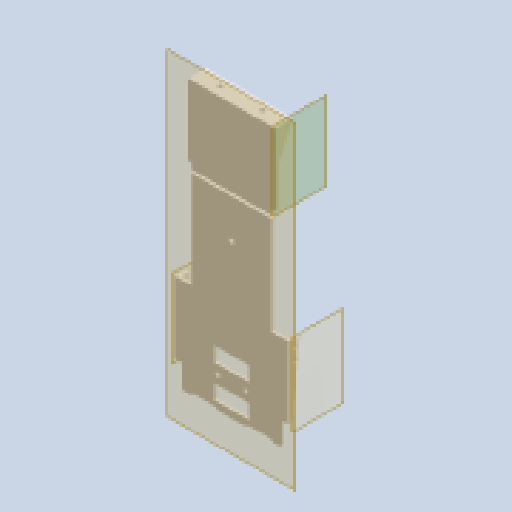
# Autodesk Inventor part: Деталь1
Saved by Autodesk Inventor 2024.2 (Build 282272000, 272)
## iProperties
Created: 2025-10-10
Part Number: Деталь1
Material: Типовые
Document SubType Name: Modeling
Designer: katya_notebook
Density: 1 g/cm^3
Appearance: По умолчанию
Author: katya_notebook
Autodesk Inventor part; units mm, degrees
ref_plane "YZ Plane" through (0, 0, 0) normal (1, 0, 0) x (0, 1, 0)
ref_plane "XZ Plane" through (0, 0, 0) normal (0, 1, 0) x (-1, 0, 0)
ref_plane "XY Plane" through (0, 0, 0) normal (0, 0, 1) x (1, 0, 0)
ref_plane "РабПлоскость1" through (46.6, -88.9135, 41) normal (0, 0, 1) x (1, 0, 0)
sketch "Эскиз1" plane through (46.6, -88.9135, 41) normal (0, 0, 1) x (1, 0, 0)
  line L0 (-9.7, 217.1229) -> (-9.7, 156.7629) projected
  line L1 (-83.5, 217.1229) -> (-9.7, 217.1229) projected
  line L2 (-83.5, 156.7629) -> (-83.5, 217.1229) projected
  line L3 (-80.1, 156.7629) -> (-83.5, 156.7629) projected
  line L4 (-80.1, 152.0768) -> (-80.1, 156.7629) projected
  line L5 (-9.7, 156.7629) -> (-13.1, 156.7629) projected
  line L6 (-13.1, 156.7629) -> (-13.1, 152.0768) projected
  line L7 (-13.1, 152.0768) -> (-80.1, 152.0768) projected
  line L8 (-13.1, 149.4521) -> (-13.1, 152.6229) projected
  line L9 (-13.1, 149.4521) -> (-13.1, 67.1229) projected
  line L10 (-80.1, 152.6229) -> (-80.1, 149.4521) projected
  line L11 (-80.1, 67.1229) -> (-80.1, 149.4521) projected
  line L12 (-13.1, 58.2834) -> (-13.1, 67.1229) projected
  line L13 (-13.1, 67.1229) -> (1.3, 67.1229) projected
  line L14 (1.3, 67.1229) -> (1.3, 6.7629) projected
  line L15 (1.3, 6.7629) -> (-4.4, 6.7629) projected
  line L16 (-4.4, 6.7629) -> (-4.4, -10.0571) projected
  arc A0 (-7.4, -13.0571) -> (-4.4, -10.0571) centre (-7.4, -10.0571) ccw projected
  line L17 (-7.4, -13.0571) -> (-10.4431, -13.0571) projected
  arc A1 (-11.7002, -12.6127) -> (-10.4431, -13.0571) centre (-10.4431, -11.0571) ccw projected
  arc A2 (-11.7002, -12.6127) -> (-16.1, -11.0571) centre (-16.1, -18.0571) ccw projected
  line L18 (-16.1, -11.0571) -> (-31.1, -11.0571) projected
  arc A3 (-31.1, -11.0571) -> (-35.4998, -12.6127) centre (-31.1, -18.0571) ccw projected
  arc A4 (-36.7569, -13.0571) -> (-35.4998, -12.6127) centre (-36.7569, -11.0571) ccw projected
  line L19 (-36.7569, -13.0571) -> (-56.4431, -13.0571) projected
  arc A5 (-57.7002, -12.6127) -> (-56.4431, -13.0571) centre (-56.4431, -11.0571) ccw projected
  arc A6 (-57.7002, -12.6127) -> (-62.1, -11.0571) centre (-62.1, -18.0571) ccw projected
  line L20 (-62.1, -11.0571) -> (-77.1, -11.0571) projected
  arc A7 (-77.1, -11.0571) -> (-81.4998, -12.6127) centre (-77.1, -18.0571) ccw projected
  arc A8 (-82.7569, -13.0571) -> (-81.4998, -12.6127) centre (-82.7569, -11.0571) ccw projected
  line L21 (-82.7569, -13.0571) -> (-85.8, -13.0571) projected
  arc A9 (-88.8, -10.0571) -> (-85.8, -13.0571) centre (-85.8, -10.0571) ccw projected
  line L22 (-88.8, -10.0571) -> (-88.8, 6.7629) projected
  line L23 (-88.8, 6.7629) -> (-94.5, 6.7629) projected
  line L24 (-94.5, 6.7629) -> (-94.5, 67.1229) projected
  line L25 (-94.5, 67.1229) -> (-80.1, 67.1229) projected
  line L26 (-83.5, 217.1229) -> (-9.7, 217.1229)
  line L27 (-9.7, 156.7629) -> (-9.7, 217.1229)
  line L28 (-9.7, 156.7629) -> (-13.1, 156.7629)
  line L29 (1.3, 67.1229) -> (-13.1, 67.1229)
  line L30 (1.3, 67.1229) -> (1.3, 6.7629)
  line L31 (-4.4, 6.7629) -> (1.3, 6.7629)
  line L32 (-4.4, 6.7629) -> (-4.4, -10.0571)
  line L33 (-16.1, -11.0571) -> (-31.1, -11.0571)
  arc A10 (-7.4, -13.0571) -> (-4.4, -10.0571) centre (-7.4, -10.0571) ccw
  arc A11 (-11.7002, -12.6127) -> (-10.4431, -13.0571) centre (-10.4431, -11.0571) ccw
  arc A12 (-11.7002, -12.6127) -> (-16.1, -11.0571) centre (-16.1, -18.0571) ccw
  line L34 (-7.4, -13.0571) -> (-10.4431, -13.0571)
  line L35 (-36.7569, -13.0571) -> (-56.4431, -13.0571)
  line L36 (-62.1, -11.0571) -> (-77.1, -11.0571)
  line L37 (-84.2784, -13.0571) -> (-85.8, -13.0571)
  line L38 (-88.8, -10.0571) -> (-88.8, 6.7629)
  line L39 (-94.5, 6.7629) -> (-88.8, 6.7629)
  line L40 (-94.5, 67.1229) -> (-94.5, 6.7629)
  line L41 (-80.1, 67.1229) -> (-94.5, 67.1229)
  line L42 (-83.5, 217.1229) -> (-83.5, 156.7629)
  line L43 (-83.5, 156.7629) -> (-80.1, 156.7629)
  arc A13 (-31.1, -11.0571) -> (-35.4998, -12.6127) centre (-31.1, -18.0571) ccw
  arc A14 (-36.7569, -13.0571) -> (-35.4998, -12.6127) centre (-36.7569, -11.0571) ccw
  arc A15 (-57.7002, -12.6127) -> (-62.1, -11.0571) centre (-62.1, -18.0571) ccw
  arc A16 (-57.7002, -12.6127) -> (-56.4431, -13.0571) centre (-56.4431, -11.0571) ccw
  arc A17 (-88.8, -10.0571) -> (-85.8, -13.0571) centre (-85.8, -10.0571) ccw
  arc A18 (-82.7569, -13.0571) -> (-81.4998, -12.6127) centre (-82.7569, -11.0571) ccw
  arc A19 (-77.1, -11.0571) -> (-81.4998, -12.6127) centre (-77.1, -18.0571) ccw
  line L44 (-82.7569, -13.0571) -> (-84.2784, -13.0571)
  line L45 (-80.1, 149.4521) -> (-13.1, 149.4521) projected
  line L46 (-80.1, 152.0768) -> (-13.1, 152.0768)
  line L47 (-13.1, 149.4521) -> (-80.1, 149.4521)
  line L48 (-13.1, 156.7629) -> (-13.1, 152.0768)
  line L49 (-13.1, 149.4521) -> (-13.1, 67.1229)
  line L50 (-80.1, 156.7629) -> (-80.1, 152.0768)
  line L51 (-80.1, 149.4521) -> (-80.1, 67.1229)
  point P0 (-46.6, 88.9135)
  constraints: 50 end point, 20 point on circle, 16 perpendicular, 10 centre point, 10 tangent, 5 collinear, 5 concentric, 4 parallel, 2 horizontal, 1 midpoint
extrude "Выдавливание1" add sketch "Эскиз1" against normal blind 2.4 contours L0 L5 L6 L7 L4 L3 L2 L1 | L9 L13 L14 L15 L16 A0 L17 A1 A2 L18 A3 A4 L19 A5 A6 L20 A7 A8 L21 A9 L22 L23 L24 L25 L11 L45
sketch "Эскиз2" plane through (46.6, -88.9135, 41) normal (0, 0, 1) x (1, 0, 0)
  line L0 (-47.85, 115.9647) -> (-47.85, 117.9647) projected
  line L1 (-47.75, 115.9647) -> (-45.45, 115.9647) projected
  line L2 (-45.45, 117.9647) -> (-47.75, 117.9647) projected
  line L3 (-45.35, 117.9647) -> (-45.35, 115.9647) projected
  line L4 (-47.85, 115.9647) -> (-45.35, 115.9647)
  line L5 (-45.35, 115.9647) -> (-45.35, 117.9647)
  line L6 (-45.35, 117.9647) -> (-47.85, 117.9647)
  line L7 (-47.85, 117.9647) -> (-47.85, 115.9647)
  line L8 (-47.85, 117.9647) -> (-45.35, 115.9647)
  line L9 (-45.35, 117.9647) -> (-47.85, 115.9647)
  line L10 (-44.6, 115.3647) -> (-48.6, 115.3647)
  line L11 (-48.6, 115.3647) -> (-48.6, 118.5647)
  line L12 (-48.6, 118.5647) -> (-44.6, 118.5647)
  line L13 (-44.6, 118.5647) -> (-44.6, 115.3647)
  line L14 (-44.6, 115.3647) -> (-48.6, 118.5647) construction
  line L15 (-48.6, 115.3647) -> (-44.6, 118.5647) construction
  point P0 (-46.6, 88.9135)
  point P1 (-46.6, 116.9647)
  dimension "d2" = 4
  dimension "d3" = 3.2
  constraints: 24 end point, 4 parallel, 3 midpoint, 2 horizontal, 2 perpendicular, 1 point on line
  measures "d2" distance of L12.end L11.end
  measures "d3" distance of L10.start L12.end
extrude "Выдавливание2" cut sketch "Эскиз2" against normal blind 2.4 contours L9 L8 L4 L1 | L0 L8 L9 | L6 L2 L9 L8 | L9 L3 L8 | L10 L11 L12 L13
ref_plane "РабПлоскость3" through (36.9, 128.2094, 0) normal (-1, 0, 0) x (0, -1, 0)
sketch "Эскиз4" plane through (36.9, 128.2094, 0) normal (-1, 0, 0) x (0, -1, 0)
  line L0 (0, 38.6) -> (60.36, 38.6) projected
  line L1 (0, 38.6) -> (0, 25.6274)
  line L2 (0, 25.6274) -> (26.6272, 38.6)
  point P0 (128.2094, 0)
  constraints: 4 end point, 1 point on line, 1 vertical
extrude "Выдавливание3" add sketch "Эскиз4" along normal up to surface (73.8 mm away)
sketch "Эскиз5" plane through (-36.9, 128.2094, 41) normal (0, 1, 0) x (1, 0, 0)
  line L0 (0, 0) -> (0, 15.3726) projected
  line L1 (73.8, 0) -> (0, 0) projected
  line L2 (0, 15.3726) -> (73.8, 15.3726)
  line L3 (73.8, 15.3726) -> (73.8, 0)
  line L4 (73.8, 0) -> (0, 0)
  line L5 (0, 0) -> (0, 15.3726)
  line L6 (36.9, 7.6863) -> (36.9, 0)
  line L7 (36.9, 7.6863) -> (78.783, 7.6863)
  circle A0 centre (54.5399, 7.6863) radius 2
  circle A1 centre (19.2601, 7.6863) radius 2
  point P0 (36.9, 41)
  dimension "d9" = 4
  constraints: 12 end point, 2 centre point, 2 horizontal, 2 parallel, 1 midpoint, 1 perpendicular, 1 point on line, 1 symmetric about line, 1 other
  measures "d9" diameter of A0
extrude "Выдавливание4" cut sketch "Эскиз5" against normal blind 100 contours A0 L7 | L7 A0 | A1
ref_plane "РабПлоскость4" through (-47.9, -82.1506, 0) normal (1, 0, 0) x (0, 1, 0)
sketch "Эскиз6" plane through (-47.9, -82.1506, 0) normal (1, 0, 0) x (0, 1, 0)
  line L0 (0, 0) -> (0, 41) projected
  circle A0 centre (9.6119, 11.875) radius 1.35 projected
  circle A1 centre (50.7481, 11.875) radius 1.35 projected
  line L1 (0, 0) -> (11.68, 0) projected
  arc A2 (48.68, 0) -> (11.68, 0) centre (30.18, 0) ccw projected
  line L2 (60.36, 0) -> (48.68, 0) projected
  line L3 (60.36, 0) -> (60.36, 41) projected
  line L4 (0, 41) -> (60.36, 41) projected
  line L5 (0, 0) -> (0, 41) projected
  line L6 (60.36, 38.6) -> (0, 38.6) projected
  line L7 (0, 38.6) -> (60.36, 31.5026)
  line L8 (60.36, 38.6) -> (60.36, 31.5026)
  line L9 (60.36, 38.6) -> (0, 38.6)
  circle A3 centre (54.6681, 35.903) radius 2 projected
  circle A4 centre (44.2207, 35.903) radius 2 projected
  point P0 (82.1506, 0)
  constraints: 6 end point, 1 collinear, 1 perpendicular, 1 point on line
extrude "Выдавливание5" add sketch "Эскиз6" along normal blind 2.5 contours L6 L3 L7 | A3 | A4
sketch "Эскиз7" plane through (47.9, -82.1506, 41) normal (1, 0, 0) x (0, 0, -1)
  line L0 (0, 60.36) -> (9.4974, 60.36) projected
  line L1 (2.4, 60.36) -> (2.4, 142.6892) projected
  line L2 (9.4974, 60.36) -> (2.4, 60.36)
  line L3 (2.4, 0) -> (9.4974, 60.36) projected
  line L4 (2.4, 60.36) -> (2.4, 0)
  line L5 (2.4, 0) -> (9.4974, 60.36)
  point P0 (41, 82.1506)
  constraints: 6 end point, 2 perpendicular, 1 collinear
extrude "Выдавливание6" add sketch "Эскиз7" against normal blind 2.5
ref_plane "РабПлоскость5" through (51, -83.4706, 0) normal (1, 0, 0) x (0, 1, 0)
sketch "Эскиз9" plane through (51, -83.4706, 0) normal (1, 0, 0) x (0, 1, 0)
  circle A0 centre (45.5407, 35.903) radius 2 projected
  circle A1 centre (55.9881, 35.903) radius 2 projected
  circle A2 centre (45.5407, 35.903) radius 2
  circle A3 centre (55.9881, 35.903) radius 2
  point P0 (83.4706, 0)
  constraints: 2 centre point, 2 coincident, 2 concentric
extrude "Выдавливание7" cut sketch "Эскиз9" against normal blind 150
sketch "Эскиз10" plane through (46.6, -88.9135, 41) normal (0, 0, 1) x (1, 0, 0)
  circle A0 centre (-58.4725, 13.1975) radius 2 projected
  circle A1 centre (-34.7275, 13.1975) radius 2 projected
  circle A2 centre (-58.4725, 13.1975) radius 2
  circle A3 centre (-34.7275, 13.1975) radius 2
  line L0 (-61.6, 33.1929) -> (-31.6, 33.1929) projected
  line L1 (-61.6, 20.6929) -> (-61.6, 33.1929) projected
  line L2 (-31.6, 20.6929) -> (-61.6, 20.6929) projected
  line L3 (-31.6, 33.1929) -> (-31.6, 20.6929) projected
  line L4 (-31.6, 20.6929) -> (-61.6, 20.6929)
  line L5 (-61.6, 20.6929) -> (-61.6, 33.1929)
  line L6 (-61.6, 33.1929) -> (-31.6, 33.1929)
  line L7 (-31.6, 33.1929) -> (-31.6, 20.6929)
  line L8 (-31.6, 20.6929) -> (-61.6, 33.1929) construction
  line L9 (-61.6, 20.6929) -> (-31.6, 33.1929) construction
  line L10 (-64.6284, 13.1975) -> (-23.2686, 13.1975)
  line L11 (-61.6, -6.7979) -> (-31.6, -6.7979)
  line L12 (-61.6, 5.7021) -> (-61.6, -6.7979)
  line L13 (-31.6, 5.7021) -> (-61.6, 5.7021)
  line L14 (-31.6, -6.7979) -> (-31.6, 5.7021)
  line L15 (-61.6, 5.7021) -> (-61.6, -6.7979)
  point P0 (-46.6, 88.9135)
  point P1 (-46.6, 26.9429)
  constraints: 24 end point, 5 symmetric about line, 2 centre point, 2 coincident, 2 concentric, 2 horizontal, 2 midpoint, 2 parallel, 1 perpendicular
extrude "Выдавливание8" cut sketch "Эскиз10" against normal blind 20
